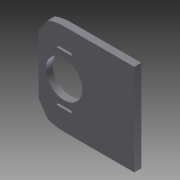
# Autodesk Inventor part: 276-2181-012 Rev1
Saved by Autodesk Inventor 2013 (Build 170138000, 138)
## iProperties
Category: Motors
Company: Autodesk Inc.
Created: 2012-01-24
Part Number: 276-2181-012 Rev1
Material: Steel
Document SubType Name: Modeling
Designer: Autodesk Inc.
Density: 7.85 g/cm^3
Catalog Web Link: http://www.vexrobotics.com/276-2181.html
Vendor: VEX
Mass: 1.17742 g
Surface Area: 3.69211 cm^2
Volume: 0.14999 cm^3
Author: Autodesk Inc.
Autodesk Inventor part; units mm, degrees
ref_plane "YZ Plane" through (0, 0, 0) normal (1, 0, 0) x (0, 1, 0)
ref_plane "XZ Plane" through (0, 0, 0) normal (0, 1, 0) x (-1, 0, 0)
ref_plane "XY Plane" through (0, 0, 0) normal (0, 0, 1) x (1, 0, 0)
sketch "Sketch1" plane through (0, 0, 0) normal (0, 0, 1) x (1, 0, 0)
  line L0 (-3.6, 4.2059) -> (-3.6, -4.2059)
  line L1 (-3.6, -4.2059) -> (-2.3111, -6.0753)
  arc A0 (-2.3111, -6.0753) -> (0, -6.5) centre (0, 0) ccw
  line L2 (0, -6.5) -> (10, -6.5)
  line L3 (10, -6.5) -> (10, 6.5)
  line L4 (10, 6.5) -> (0, 6.5)
  arc A1 (0, 6.5) -> (-2.3111, 6.0753) centre (0, 0) ccw
  line L5 (-2.3111, 6.0753) -> (-3.6, 4.2059)
  circle A2 centre (0, 0) radius 2.6
  constraints: 12 end point, 4 point on circle, 3 centre point
extrude "Extrusion1" add sketch "Sketch1" against normal blind 0.9906
sketch "Sketch2" plane through (0, 0, 0) normal (0, 0, 1) x (1, 0, 0)
  line L0 (-1.0714, 3.7) -> (1.0714, 3.7) projected
  line L1 (-1.0714, 3.4) -> (-1.0714, 3.7) projected
  line L2 (1.0714, 3.4) -> (-1.0714, 3.4) projected
  line L3 (1.0714, 3.7) -> (1.0714, 3.4) projected
  line L4 (-1.0714, -3.4) -> (1.0714, -3.4) projected
  line L5 (-1.0714, -3.7) -> (-1.0714, -3.4) projected
  line L6 (1.0714, -3.7) -> (-1.0714, -3.7) projected
  line L7 (1.0714, -3.4) -> (1.0714, -3.7) projected
extrude "Extrusion2" cut sketch "Sketch2" against normal up to next
body "Solid1"
